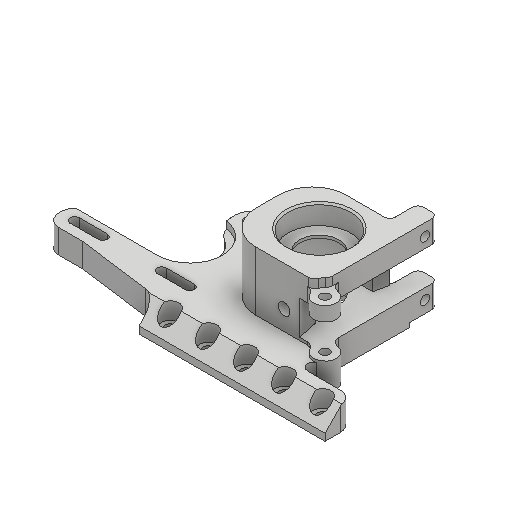
# Autodesk Inventor part: 3DP_ABS_Extruder_Body
Saved by Autodesk Inventor 2026.1 (Build 301233000, 233)
## iProperties
Created: 2016-01-22
Part Number: 3DP_ABS_Extruder_Body
Material: Ogólny
Document SubType Name: Modeling
Designer: Andrzej
Density: 1 g/cm^3
Appearance: Domyślna
Mass: 33.8707 g
Surface Area: 154.529 cm^2
Volume: 33.8707 cm^3
Author: Andrzej
Autodesk Inventor part; units mm, degrees
ref_plane "YZ Plane" through (0, 0, 0) normal (1, 0, 0) x (0, 1, 0)
ref_plane "XZ Plane" through (0, 0, 0) normal (0, 1, 0) x (-1, 0, 0)
ref_plane "XY Plane" through (0, 0, 0) normal (0, 0, 1) x (1, 0, 0)
sketch "Szkic1" plane through (0, 0, 0) normal (0, 0, 1) x (1, 0, 0)
  line L0 (3.1632, -2.8776) -> (69.1632, -2.8776)
  line L1 (69.1632, -2.8776) -> (69.1632, 7.1224)
  line L2 (3.1632, -2.8776) -> (3.1632, 7.1224)
  line L3 (3.1632, 7.1224) -> (69.1632, 7.1224)
  line L4 (3.1632, 7.1224) -> (-39.8368, 7.1224)
  line L5 (-39.8368, 7.1224) -> (-39.8368, 17.1224)
  line L6 (12.1632, 17.1224) -> (12.1632, 47.1224)
  line L7 (12.1632, 47.1224) -> (-7.8368, 47.1224)
  line L8 (-7.8368, 47.1224) -> (-7.8368, 17.1224)
  line L9 (-39.8368, 17.1224) -> (-7.8368, 17.1224)
  line L10 (12.1632, 7.1224) -> (12.1632, 17.1224)
  line L11 (-34.7368, 12.1224) -> (-24.7368, 12.1224) construction
  line L12 (-34.7368, 10.4724) -> (-24.7368, 10.4724)
  line L13 (-24.7368, 13.7724) -> (-34.7368, 13.7724)
  arc A0 (-34.7368, 13.7724) -> (-34.7368, 10.4724) centre (-34.7368, 12.1224) ccw
  arc A1 (-24.7368, 10.4724) -> (-24.7368, 13.7724) centre (-24.7368, 12.1224) ccw
  line L14 (-3.8368, 43.0224) -> (6.1632, 43.0224) construction
  line L15 (-3.8368, 41.3724) -> (6.1632, 41.3724)
  line L16 (6.1632, 44.6724) -> (-3.8368, 44.6724)
  arc A2 (-3.8368, 44.6724) -> (-3.8368, 41.3724) centre (-3.8368, 43.0224) ccw
  arc A3 (6.1632, 41.3724) -> (6.1632, 44.6724) centre (6.1632, 43.0224) ccw
  line L17 (-3.8368, 12.1224) -> (6.1632, 12.1224) construction
  line L18 (-3.8368, 10.4724) -> (6.1632, 10.4724)
  line L19 (6.1632, 13.7724) -> (-3.8368, 13.7724)
  arc A4 (-3.8368, 13.7724) -> (-3.8368, 10.4724) centre (-3.8368, 12.1224) ccw
  arc A5 (6.1632, 10.4724) -> (6.1632, 13.7724) centre (6.1632, 12.1224) ccw
  circle A6 centre (32.1632, 32.1224) radius 4.25
  circle A7 centre (32.1632, 32.1224) radius 11.125
  line L20 (12.1632, 47.1224) -> (49.1632, 47.1224)
  line L21 (49.1632, 47.1224) -> (49.1632, 7.1224)
  circle A8 centre (32.1632, 32.1224) radius 7
  point P0 (0, 0)
  point P1 (9.1632, 2.1224)
  point P2 (22.6632, 2.1224)
  point P3 (36.1632, 2.1224)
  point P4 (49.6632, 2.1224)
  point P5 (63.1632, 2.1224)
  point P6 (-29.7368, 12.1224)
  point P7 (1.1632, 12.1224)
  point P8 (1.1632, 43.0224)
  point P9 (-15.7868, 27.5724)
  dimension "d0" = 66
  dimension "d1" = 10
  dimension "d6" = 13.5
  dimension "d7" = 13.5
  dimension "d8" = 13.5
  dimension "d9" = 13.5
  dimension "d10" = 6
  dimension "d11" = 5
  dimension "d23" = 43
  dimension "d28" = 37
  dimension "d44" = 5
  dimension "d45" = 5
  dimension "d47" = 30.9
  dimension "d50" = 30
  dimension "d51" = 11
  dimension "d53" = 11
  dimension "d54" = 30.9
  dimension "d93" = 15.45
  dimension "d95" = 20
  dimension "d96" = 57
  dimension "d97" = 9
  dimension "d100" = 5
  dimension "d101" = 3.3
  dimension "d102" = 5
  dimension "d103" = 3.3
  dimension "d104" = 5
  dimension "d105" = 3.3
  dimension "d108" = 8.5
  dimension "d110" = 25
  dimension "d111" = 22.25
  dimension "d112" = 37
  dimension "d253" = 14
  constraints: 50 end point, 12 point on circle, 12 tangent, 9 centre point, 5 perpendicular, 4 horizontal, 4 parallel, 3 midpoint, 3 point on line, 3 vertical, 2 coincident
  measures "d0" distance of L0.start L0.end
  measures "d1" distance of L0.end L1.end
  measures "d6" distance of point (22.663, 2.122) point (9.163, 2.122)
  measures "d7" distance of point (22.663, 2.122) point (36.163, 2.122)
  measures "d8" distance of point (36.163, 2.122) point (49.663, 2.122)
  measures "d9" distance of point (49.663, 2.122) point (63.163, 2.122)
  measures "d10" distance from line of L2 point (9.163, 2.122)
  measures "d11" distance from line of L0 point (9.163, 2.122)
  measures "d23" distance of L2.end L4.end
  measures "d28" distance from line of L1 point (32.163, 32.122)
  measures "d44" distance from line of L4 point (-29.737, 12.122)
  measures "d45" distance from line of L3 point (1.163, 12.122)
  measures "d47" distance of point (1.163, 12.122) point (-29.737, 12.122)
  measures "d50" distance of L6.start L6.end
  measures "d51" distance from line of point (1.163, 12.122) L6
  measures "d53" distance from line of L6 point (1.163, 43.022)
  measures "d54" distance of point (1.163, 43.022) point (1.163, 12.122)
  measures "d93" vertical distance of point (-15.787, 27.572) point (-29.737, 12.122)
  measures "d95" distance of L6.end L7.end
  measures "d96" distance between parallel lines of L1 L10
  measures "d97" distance from line of L8 point (1.163, 12.122)
  measures "d100" distance of point (-29.737, 12.122) L11.end
  measures "d101" diameter of A1
  measures "d102" distance of point (1.163, 43.022) L14.end
  measures "d103" diameter of A3
  measures "d104" distance of point (1.163, 12.122) L17.end
  measures "d105" diameter of A5
  measures "d108" diameter of A6
  measures "d110" distance from line of L3 A6.centre
  measures "d111" diameter of A7
  measures "d112" distance of L6.end L20.end
  measures "d253" diameter of A8
extrude "Wyciągnięcie proste6" add sketch "Szkic1" along normal blind 8.5 contours L2 L3 L1 L0 | L4 L5 L9 L8 L7 L6 L10 L3 | L10 L6 L20 L21 L3 | A7 | A8
extrude "Wyciągnięcie proste7" cut sketch "Szkic1" along normal blind 7 contours A7 | A8
hole "Otwór3" at (9.1632, 2.1224, 0) at (22.6632, 2.1224, 0) at (36.1632, 2.1224, 0) at (49.6632, 2.1224, 0) at (63.1632, 2.1224, 0) at (32.1632, 32.1224, 0) at (-29.7368, 12.1224, 0) at (1.1632, 12.1224, 0) at (1.1632, 43.0224, 0) at (-15.7868, 27.5724, 0) direction (0, 0, 1) diameter 3.25 end through all
chamfer "Faza3" distance 30 distance2 4 1 edges at (3.1632, 7.1224, 4.25) measured on face at (-25.5035, 7.1224, 5.6667)
sketch "Szkic4" plane through (0, 0, 8.5) normal (0, 0, 1) x (1, 0, 0)
  arc A0 (6.1632, 41.3724) -> (6.1632, 44.6724) centre (6.1632, 43.0224) ccw projected
  arc A1 (6.1632, 41.3724) -> (6.1632, 44.6724) centre (6.1632, 43.0224) ccw projected
  arc A2 (6.1632, 10.4724) -> (6.1632, 13.7724) centre (6.1632, 12.1224) ccw projected
  arc A3 (6.1632, 10.4724) -> (6.1632, 13.7724) centre (6.1632, 12.1224) ccw projected
  line L0 (-31.6302, 7.1137) -> (58.7822, 7.1137)
  line L1 (14.6632, 7.1137) -> (14.6632, 47.1224)
  line L2 (49.1632, 47.1224) -> (-7.8368, 47.1224) projected
  circle A4 centre (32.1632, 32.1224) radius 4.25 projected
  line L3 (69.1632, 7.1224) -> (49.1632, 7.1224) projected
  line L4 (49.1632, 7.1224) -> (49.1632, 47.1224) projected
  line L5 (49.1632, 47.1224) -> (-7.8368, 47.1224) projected
  line L6 (-7.8368, 47.1224) -> (-7.8368, 17.1224) projected
  line L7 (-7.8368, 17.1224) -> (-39.8368, 17.1224) projected
  line L8 (-39.8368, 17.1224) -> (-39.8368, 7.1224) projected
  line L9 (-39.8368, 7.1224) -> (-26.8368, 7.1224) projected
  line L10 (3.1632, 3.1224) -> (-26.8368, 7.1224) projected
  line L11 (3.1632, 3.1224) -> (3.1632, -2.8776) projected
  line L12 (3.1632, -2.8776) -> (69.1632, -2.8776) projected
  line L13 (69.1632, -2.8776) -> (69.1632, 7.1224) projected
  arc A5 (-34.7368, 13.7724) -> (-34.7368, 10.4724) centre (-34.7368, 12.1224) ccw projected
  line L14 (-34.7368, 13.7724) -> (-24.7368, 13.7724) projected
  arc A6 (-24.7368, 10.4724) -> (-24.7368, 13.7724) centre (-24.7368, 12.1224) ccw projected
  line L15 (-24.7368, 10.4724) -> (-34.7368, 10.4724) projected
  arc A7 (-3.8368, 44.6724) -> (-3.8368, 41.3724) centre (-3.8368, 43.0224) ccw projected
  line L16 (-3.8368, 44.6724) -> (6.1632, 44.6724) projected
  arc A8 (6.1632, 41.3724) -> (6.1632, 44.6724) centre (6.1632, 43.0224) ccw projected
  line L17 (6.1632, 41.3724) -> (-3.8368, 41.3724) projected
  arc A9 (-3.8368, 13.7724) -> (-3.8368, 10.4724) centre (-3.8368, 12.1224) ccw projected
  line L18 (-3.8368, 13.7724) -> (6.1632, 13.7724) projected
  arc A10 (6.1632, 10.4724) -> (6.1632, 13.7724) centre (6.1632, 12.1224) ccw projected
  line L19 (6.1632, 10.4724) -> (-3.8368, 10.4724) projected
  circle A11 centre (32.1632, 32.1224) radius 4.25 projected
  circle A12 centre (49.6632, 2.1224) radius 1.625 projected
  circle A13 centre (22.6632, 2.1224) radius 1.625 projected
  circle A14 centre (9.1632, 2.1224) radius 1.625 projected
  circle A15 centre (36.1632, 2.1224) radius 1.625 projected
  circle A16 centre (63.1632, 2.1224) radius 1.625 projected
  line L20 (14.6632, 15.1224) -> (49.1632, 15.1224)
  line L21 (49.1632, 11.6224) -> (49.1632, 35.1224) projected
  line L22 (49.1632, 15.1224) -> (49.1632, 35.1224)
  line L23 (49.1632, 47.1224) -> (-7.8368, 47.1224) projected
  line L24 (14.6632, 47.1224) -> (49.1632, 47.1224)
  line L25 (49.1632, 47.1224) -> (49.1632, 15.1224)
  point P0 (0, 0)
  point P1 (37.1632, 47.1224)
  point P2 (0.6632, 47.1224)
  dimension "d127" = 8.5
  dimension "d129" = 32
  dimension "d133" = 34.5
  constraints: 12 end point, 4 point on line, 2 collinear, 1 horizontal, 1 perpendicular, 1 vertical
  measures "d127" distance from line of L1 A0.centre
  measures "d129" distance between parallel lines of L20 L2
  measures "d133" distance between parallel lines of L4 L1
extrude "Wyciągnięcie proste8" add sketch "Szkic4" along normal blind 1 contours L1 L2 L4 L20
fillet "Zaokrąglenie3" radius 4.5 6 edges at (-39.8368, 17.1224, 4.25) (-7.8368, 17.1224, 4.25) (-7.8368, 47.1224, 4.25) (49.1632, 7.1224, 4.25) (69.1632, 7.1224, 4.25) (-39.8368, 7.1224, 4.25)
sketch "Szkic5" plane through (0, 0, 9.5) normal (0, 0, 1) x (1, 0, 0)
  circle A0 centre (32.1632, 32.1224) radius 4.25 projected
  line L0 (14.6632, 47.1224) -> (14.6632, 15.1224) projected
  line L1 (14.6632, 15.1224) -> (49.1632, 15.1224) projected
  line L2 (49.1632, 15.1224) -> (49.1632, 47.1224) projected
  line L3 (49.1632, 47.1224) -> (14.6632, 47.1224) projected
  line L4 (14.6632, 15.1224) -> (49.1632, 15.1224) projected
  line L5 (42.1632, 42.1224) -> (42.1632, 47.1224)
  line L6 (42.1632, 22.1224) -> (42.1632, 15.1224)
  line L7 (42.1632, 47.1224) -> (14.6632, 47.1224)
  line L8 (14.6632, 47.1224) -> (14.6632, 15.1224) projected
  line L9 (14.6632, 15.1224) -> (14.6632, 47.1224)
  line L10 (14.6632, 15.1224) -> (42.1632, 15.1224)
  arc A1 (47.1632, 15.1224) -> (49.1632, 18.5865) centre (51.1632, 15.1224) ccw
  arc A2 (32.1632, 42.1224) -> (32.1632, 22.1224) centre (32.1632, 32.1224) ccw
  line L11 (32.1632, 42.1224) -> (42.1632, 42.1224)
  line L12 (32.1632, 22.1224) -> (42.1632, 22.1224)
  point P0 (0, 0)
  point P1 (49.1632, 26.9954)
  point P2 (49.1632, 19.2494)
  dimension "d140" = 7
  dimension "d149" = 9
  dimension "d150" = 0
  dimension "d162" = 8
  dimension "d163" = 7
  dimension "d164" = 20
  constraints: 14 end point, 5 point on line, 4 perpendicular, 4 point on circle, 2 centre point, 2 coincident, 2 tangent, 1 collinear, 1 parallel, 1 vertical
  measures "d140" distance between parallel lines of L2 L6
  measures "d149" distance from line of point (51.163, 15.122) L6
  measures "d150" distance from line of L1 point (51.163, 15.122)
  measures "d162" diameter of A1
  measures "d163" distance between parallel lines of L2 L5
  measures "d164" diameter of A2
extrude "Wyciągnięcie proste9" add sketch "Szkic5" along normal blind 12 contours L3 L5 L11 A2 L12 L6 L1 L0
extrude "Wyciągnięcie proste13" add sketch "Szkic5" against normal blind 9.5 contours L1 L2 A1
hole "Otwór4" at (51.1632, 15.1224, 9.5) direction (0, 0, -1) diameter 3.25 end through all
sketch "Szkic8" plane through (0, 0, 8.5) normal (0, 0, 1) x (1, 0, 0)
  line L0 (6.1632, 41.3724) -> (-3.8368, 41.3724) projected
  arc A0 (-3.8368, 44.6724) -> (-3.8368, 41.3724) centre (-3.8368, 43.0224) ccw projected
  line L1 (-3.8368, 44.6724) -> (6.1632, 44.6724) projected
  arc A1 (6.1632, 41.3724) -> (6.1632, 44.6724) centre (6.1632, 43.0224) ccw projected
  line L2 (-3.8368, 13.7724) -> (6.1632, 13.7724) projected
  arc A2 (-3.8368, 13.7724) -> (-3.8368, 10.4724) centre (-3.8368, 12.1224) ccw projected
  line L3 (6.1632, 10.4724) -> (-3.8368, 10.4724) projected
  arc A3 (6.1632, 10.4724) -> (6.1632, 13.7724) centre (6.1632, 12.1224) ccw projected
  arc A4 (-24.7368, 10.4724) -> (-24.7368, 13.7724) centre (-24.7368, 12.1224) ccw projected
  arc A5 (-9.2868, 16.0724) -> (-7.8368, 38.9807) centre (-9.2868, 27.5724) ccw
  circle A6 centre (63.1632, 2.1224) radius 1.625 projected
  circle A7 centre (36.1632, 2.1224) radius 1.625 projected
  circle A8 centre (9.1632, 2.1224) radius 1.625 projected
  circle A9 centre (22.6632, 2.1224) radius 1.625 projected
  circle A10 centre (49.6632, 2.1224) radius 1.625 projected
  arc A11 (-3.8368, 13.7724) -> (-3.8368, 10.4724) centre (-3.8368, 12.1224) ccw projected
  line L4 (-3.8368, 13.7724) -> (6.1632, 13.7724) projected
  arc A12 (6.1632, 10.4724) -> (6.1632, 13.7724) centre (6.1632, 12.1224) ccw projected
  line L5 (6.1632, 10.4724) -> (-3.8368, 10.4724) projected
  arc A13 (-3.8368, 44.6724) -> (-3.8368, 41.3724) centre (-3.8368, 43.0224) ccw projected
  line L6 (-3.8368, 44.6724) -> (6.1632, 44.6724) projected
  arc A14 (6.1632, 41.3724) -> (6.1632, 44.6724) centre (6.1632, 43.0224) ccw projected
  line L7 (6.1632, 41.3724) -> (-3.8368, 41.3724) projected
  arc A15 (-34.7368, 13.7724) -> (-34.7368, 10.4724) centre (-34.7368, 12.1224) ccw projected
  line L8 (-34.7368, 13.7724) -> (-24.7368, 13.7724) projected
  arc A16 (-24.7368, 10.4724) -> (-24.7368, 13.7724) centre (-24.7368, 12.1224) ccw projected
  line L9 (-24.7368, 10.4724) -> (-34.7368, 10.4724) projected
  arc A17 (47.1632, 15.1224) -> (49.1632, 11.6583) centre (51.1632, 15.1224) ccw projected
  line L10 (47.1632, 15.1224) -> (14.6632, 15.1224) projected
  line L11 (14.6632, 15.1224) -> (14.6632, 47.1224) projected
  line L12 (14.6632, 47.1224) -> (-3.3368, 47.1224) projected
  arc A18 (-3.3368, 47.1224) -> (-7.8368, 42.6224) centre (-3.3368, 42.6224) ccw projected
  line L13 (-7.8368, 42.6224) -> (-7.8368, 21.6224) projected
  arc A19 (-12.3368, 17.1224) -> (-7.8368, 21.6224) centre (-12.3368, 21.6224) ccw projected
  line L14 (-12.3368, 17.1224) -> (-35.3368, 17.1224) projected
  arc A20 (-35.3368, 17.1224) -> (-39.8368, 12.6224) centre (-35.3368, 12.6224) ccw projected
  line L15 (-39.8368, 12.6224) -> (-39.8368, 11.6224) projected
  arc A21 (-39.8368, 11.6224) -> (-35.3368, 7.1224) centre (-35.3368, 11.6224) ccw projected
  line L16 (-35.3368, 7.1224) -> (-26.8368, 7.1224) projected
  line L17 (3.1632, 3.1224) -> (-26.8368, 7.1224) projected
  line L18 (3.1632, 3.1224) -> (3.1632, -2.8776) projected
  line L19 (3.1632, -2.8776) -> (69.1632, -2.8776) projected
  line L20 (69.1632, -2.8776) -> (69.1632, 2.6224) projected
  arc A22 (69.1632, 2.6224) -> (64.6632, 7.1224) centre (64.6632, 2.6224) ccw projected
  line L21 (64.6632, 7.1224) -> (53.6632, 7.1224) projected
  arc A23 (49.1632, 11.6224) -> (53.6632, 7.1224) centre (53.6632, 11.6224) ccw projected
  line L22 (49.1632, 11.6224) -> (49.1632, 11.6583) projected
  line L23 (-9.2868, 16.0724) -> (-38.226, 16.0724)
  circle A24 centre (-9.2868, 27.5724) radius 9
  point P0 (0, 0)
  dimension "d165" = 15.45
  dimension "d166" = 15.45
  dimension "d167" = 23
  dimension "d172" = 18
  constraints: 3 point on circle, 2 centre point, 2 coincident, 2 end point, 1 horizontal, 1 point on line
  measures "d165" horizontal distance of point (-9.287, 27.572) A1.centre
  measures "d166" horizontal distance of A4.centre point (-9.287, 27.572)
  measures "d167" diameter of A5
  measures "d172" diameter of A24
extrude "Wyciągnięcie proste15" cut sketch "Szkic8" against normal blind 2.5 contours L23 A20 L14 A19 A24 L13 A5 | A24 A19 L13 picked at (-7.1612, 31.317)
extrude "Wyciągnięcie proste16" cut sketch "Szkic8" against normal up to surface (8.5 mm away) contours A24 A19 L13 | L13 A19 A24
sketch "Szkic9" plane through (49.1632, 47.1224, 9.5) normal (0, 1, 0) x (1, 0, 0)
  line L0 (-52.5, 1) -> (-52.5, 9.5) projected
  line L1 (-34.5, 1) -> (-52.5, 1) projected
  line L2 (-34.5, 1) -> (-34.5, -12) projected
  line L3 (-7, 0) -> (-7, -12) projected
  line L4 (0, 0) -> (-7, 0) projected
  line L5 (0, 9.5) -> (0, 0) projected
  line L6 (0, 9.5) -> (-52.5, 9.5) projected
  line L7 (-7, 0) -> (-17, 0) projected
  line L8 (-7, -12) -> (-34.5, -12) projected
  point P0 (-49.1632, 9.5)
  point P1 (-12.475, -6)
  dimension "d175" = 5.475
  dimension "d205" = 6
  measures "d175" distance from line of L3 point (-12.475, -6)
  measures "d205" distance from line of L7 point (-12.475, -6)
hole "Otwór5" at (36.6882, 47.1224, 15.5) direction (0, -1, 0) diameter 4.2 end through all
sketch "Szkic10" plane through (0, 0, 8.5) normal (0, 0, 1) x (1, 0, 0)
  circle A0 centre (9.1632, 2.1224) radius 1.625 projected
  circle A1 centre (22.6632, 2.1224) radius 1.625 projected
  circle A2 centre (36.1632, 2.1224) radius 1.625 projected
  circle A3 centre (49.6632, 2.1224) radius 1.625 projected
  circle A4 centre (63.1632, 2.1224) radius 1.625 projected
  circle A5 centre (9.1632, 2.1224) radius 3.15
  circle A6 centre (22.6632, 2.1224) radius 3.15
  circle A7 centre (36.1632, 2.1224) radius 3.15
  circle A8 centre (49.6632, 2.1224) radius 3.15
  circle A9 centre (63.1632, 2.1224) radius 3.15
  point P0 (0, 0)
  dimension "d185" = 6.3
  dimension "d186" = 6.3
  dimension "d187" = 6.3
  dimension "d188" = 6.3
  dimension "d189" = 6.3
  constraints: 5 centre point, 5 coincident
  measures "d185" diameter of A5
  measures "d186" diameter of A6
  measures "d187" diameter of A7
  measures "d188" diameter of A8
  measures "d189" diameter of A9
extrude "Wyciągnięcie proste17" cut sketch "Szkic10" against normal blind 6
chamfer "Faza4" distance 6 angle 45 1 edges at (36.1632, -2.8776, 8.5)
chamfer "Faza5" distance 7 distance2 1.5 1 edges at (42.1632, 22.1224, 15.5) measured on face at (42.1632, 17.4558, 13.5)
chamfer "Faza6" distance 1 distance2 5 1 edges at (42.1632, 42.1224, 15.5) measured on face at (41.0331, 42.1224, 15.5844)
sketch "Szkic11" plane through (0, 0, 21.5) normal (0, 0, 1) x (1, 0, 0)
  line L0 (49.1632, 47.1224) -> (42.1632, 47.1224) projected
  line L1 (14.6632, 15.1224) -> (42.1632, 15.1224) projected
  line L2 (49.1632, 47.1224) -> (14.6632, 47.1224)
  line L3 (14.6632, 47.1224) -> (14.6632, 15.1224)
  line L4 (14.6632, 15.1224) -> (47.1632, 15.1224)
  line L5 (49.1632, 18.5865) -> (49.1632, 47.1224)
  circle A0 centre (51.1632, 15.1224) radius 4
  point P0 (0, 0)
  dimension "d115" = 3.25
  dimension "d117" = 4
  dimension "d118" = 2
  dimension "d120" = 8
  dimension "d206" = 2
  dimension "d207" = 8
  constraints: 8 end point, 2 parallel, 2 point on circle, 1 centre point, 1 coincident, 1 horizontal, 1 perpendicular
  measures "d206" distance from line of L5 point (51.163, 15.122)
  measures "d207" diameter of A0
extrude "Wyciągnięcie proste19" add sketch "Szkic11" along normal blind 8 contours L5 A0 L4 L1 L3 L2 L0
extrude "Wyciągnięcie proste20" add sketch "Szkic11" along normal blind 5 contours A0
hole "Otwór6" at (51.1632, 15.1224, 21.5) direction (0, 0, 1) diameter 3.25 end through all
sketch "Szkic12" plane through (0, 0, 0) normal (0, 0, -1) x (-1, 0, 0)
  circle A0 centre (-51.1632, 15.1224) radius 1.625 projected
  line L0 (-49.4023, 18.1724) -> (-47.6414, 15.1224)
  line L1 (-47.6414, 15.1224) -> (-49.4023, 12.0724)
  line L2 (-49.4023, 12.0724) -> (-52.9241, 12.0724)
  line L3 (-52.9241, 12.0724) -> (-54.685, 15.1224)
  line L4 (-54.685, 15.1224) -> (-52.9241, 18.1724)
  line L5 (-52.9241, 18.1724) -> (-49.4023, 18.1724)
  point P0 (0, 0)
  point P1 (-51.1632, 18.1724)
  constraints: 12 end point, 1 midpoint, 13 other
extrude "Wyciągnięcie proste21" cut sketch "Szkic12" against normal blind 5
fillet "Zaokrąglenie4" radius 3 4 edges at (47.1632, 15.1224, 24) (49.1632, 18.5865, 24) (49.1632, 18.5865, 4.75) (47.1632, 15.1224, 9)
fillet "Zaokrąglenie5" radius 2 1 edges at (49.1632, 11.6583, 4.25)
sketch "Szkic13" plane through (0, 0, 29.5) normal (0, 0, 1) x (1, 0, 0)
  circle A0 centre (32.1632, 32.1224) radius 11.125 projected
  circle A1 centre (32.1632, 32.1224) radius 4.25 projected
  circle A2 centre (32.1632, 32.1224) radius 7
  point P0 (0, 0)
  dimension "d256" = 14
  constraints: 1 centre point, 1 coincident
  measures "d256" diameter of A2
extrude "Wyciągnięcie proste22" cut sketch "Szkic13" against normal blind 8 contours A1
extrude "Wyciągnięcie proste23" cut sketch "Szkic13" against normal blind 7 contours A0 | A2
sketch "Szkic14" plane through (49.1632, 47.1224, 9.5) normal (0, 1, 0) x (1, 0, 0)
  line L0 (0, -20) -> (-2, -20) projected
  line L1 (0, -12) -> (0, -17) projected
  line L2 (0, -20) -> (0, -12)
  line L3 (-8.5, -12) -> (-7, -12) projected
  line L4 (0, -12) -> (-7, -12)
  line L5 (-7, -12) -> (-7, -20)
  line L6 (-8.5, -12) -> (-17, -12) projected
  line L7 (-7, -20) -> (0, -20)
  line L8 (0, 8) -> (-7, 8)
  line L9 (-7, 0) -> (-8.5, 0) projected
  line L10 (-7, 8) -> (-7, 0)
  line L11 (0, 0) -> (2.5714, 0) projected
  line L12 (-7, 0) -> (0, 0)
  line L13 (0, 0) -> (0, 8)
  dimension "d266" = 7
  dimension "d267" = 7
  dimension "d268" = 28
  constraints: 16 end point, 3 perpendicular, 2 collinear, 1 horizontal, 1 vertical
  measures "d266" distance of L1.start L3.end
  measures "d267" distance of L8.start L8.end
  measures "d268" distance between parallel lines of L7 L8
extrude "Wyciągnięcie proste24" add sketch "Szkic14" along normal blind 10
fillet "Zaokrąglenie8" radius 2.5 2 edges at (49.1632, 18.5865, 28) (47.1632, 15.1224, 28)
extrude "Wyciągnięcie proste26" cut sketch "Szkic1" along normal blind 10 contours A8
extrude "Wyciągnięcie proste27" cut sketch "Szkic13" against normal blind 8 contours A2
chamfer "Faza7" distance 0.6 angle 45 2 edges at (21.0382, 32.1224, 29.5) (21.0382, 32.1224, 0)
sketch "Szkic16" plane through (42.1632, 47.1224, 1.5) normal (-1, 0, 0) x (0, 0, 1)
  line L0 (8, 0) -> (0, 0) projected
  line L1 (8, 0) -> (8, 10) projected
  line L2 (0, 10) -> (8, 10) projected
  line L3 (0, 0) -> (0, 10) projected
  line L4 (28, 0) -> (20, 0) projected
  line L5 (28, 0) -> (28, 10) projected
  line L6 (20, 10) -> (28, 10) projected
  line L7 (20, 0) -> (20, 10) projected
  line L8 (20.85, 7.1743) -> (23.75, 8.8486)
  line L9 (23.75, 8.8486) -> (26.65, 7.1743)
  line L10 (26.65, 7.1743) -> (26.65, 3.8257)
  line L11 (26.65, 3.8257) -> (23.75, 2.1514)
  line L12 (23.75, 2.1514) -> (20.85, 3.8257)
  line L13 (20.85, 3.8257) -> (20.85, 7.1743)
  line L14 (7.15, 3.8257) -> (4.25, 2.1514)
  line L15 (4.25, 2.1514) -> (1.35, 3.8257)
  line L16 (1.35, 3.8257) -> (1.35, 7.1743)
  line L17 (1.35, 7.1743) -> (4.25, 8.8486)
  line L18 (4.25, 8.8486) -> (7.15, 7.1743)
  line L19 (7.15, 7.1743) -> (7.15, 3.8257)
  point P0 (-1.5, -47.1224)
  point P1 (4.25, 5.5)
  point P2 (23.75, 5.5)
  point P3 (23.75, 5.5)
  point P4 (20.85, 5.5)
  point P5 (4.25, 5.5)
  point P6 (7.15, 5.5)
  dimension "d269" = 4.25
  dimension "d270" = 5.5
  dimension "d271" = 4.25
  dimension "d272" = 5.5
  dimension "d284" = 2.1514
  dimension "d285" = 2.1514
  constraints: 24 end point, 2 midpoint, 26 other
  measures "d269" distance from line of L5 point (23.75, 5.5)
  measures "d270" distance from line of L4 point (23.75, 5.5)
  measures "d271" distance from line of L3 point (4.25, 5.5)
  measures "d272" distance from line of L0 point (4.25, 5.5)
  measures "d284" distance from line of L0 L14.end
  measures "d285" distance from line of L4 L11.end
extrude "Wyciągnięcie proste28" cut sketch "Szkic16" against normal blind 3 contours L8 L9 L10 L11 L12 L13 | L14 L15 L16 L17 L18 L19
hole "Otwór8" at (42.1632, 52.6224, 5.75) at (42.1632, 52.6224, 25.25) direction (1, 0, 0) diameter 3.25 end through all
fillet "Zaokrąglenie9" radius 2 6 edges at (49.1632, 57.1224, 25.5) (42.1632, 57.1224, 25.5) (42.1632, 47.1224, 25.5) (49.1632, 57.1224, 5.5) (42.1632, 57.1224, 5.5) (42.1632, 47.1224, 5.5)
fillet "Zaokrąglenie10" radius 12 2 edges at (14.6632, 47.1224, 19) (14.6632, 15.1224, 19)
fillet "Zaokrąglenie11" radius 6 2 edges at (-7.8368, 36.4549, 3) (-9.0246, 18.5763, 3)
fillet "Zaokrąglenie11" radius 5 1 edges at (3.1632, 3.1224, 4.25)
equation "\"d7\" = d6"
equation "\"d8\" = d6"
equation "\"d9\" = d6"
equation "\"d11\" = 0.5 * d1"
